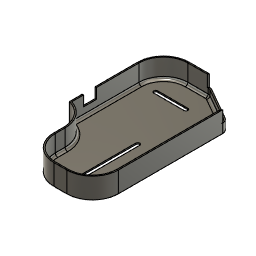
case (Autodesk Fusion 360 design; units mm, degrees)
Autodesk Fusion 360 part; units mm, degrees
note: some values were not read from the file. Chosen so that the rebuilt part matches the saved one: a direction.
sketch "Sketch1" plane through (0, 0, 0) normal (0, 1, 0) x (1, 0, 0)
  line L0 (-0.1777, 0.064) -> (49.8223, 0.064)
  line L1 (49.8223, 0.064) -> (49.8223, -119.936)
  line L2 (49.8223, -119.936) -> (-0.1777, -119.936)
  line L3 (-0.1777, -119.936) -> (-0.1777, 0.064)
  line L4 (-0.1777, 0.064) -> (-15.1777, 0.064)
  line L5 (-15.1777, 0.064) -> (-15.1777, -72.936)
  line L6 (-15.1777, -72.936) -> (-0.1777, -72.936)
  line L7 (-0.1777, -72.936) -> (-0.1777, 0.064)
  dimension "d1" = 50
  dimension "d2" = 120
  dimension "d3" = 15
  dimension "d4" = 73
  constraint horizontal L0
  constraint vertical L1
  constraint horizontal L2
  constraint vertical L3
  constraint horizontal L4
  constraint vertical L5
  constraint horizontal L6
  constraint vertical L7
  measures "d1" distance of L0.start L0.end
  measures "d2" distance of L0.start L2.end
  measures "d3" distance of L0.start L4.end
  measures "d4" distance of L0.start L6.end
extrude "Extrude1" add sketch "Sketch1" along normal blind 2
fillet "Fillet1" radius 20 4 edges at (-0.1777, 1, 72.936) (-0.1777, 1, 119.936) (49.8223, 1, 119.936) (-15.1777, 1, -0.064)
sketch "Sketch2" plane through (0, 2, 0) normal (0, 1, 0) x (-1, 0, 0)
  arc A0 (-4.8223, -0.064) -> (15.1777, 19.936) centre (-4.8223, 19.936) ccw
  line L0 (15.1777, 19.936) -> (15.1777, 72.936)
  arc A1 (0.1777, 92.3009) -> (15.1777, 72.936) centre (20.1777, 92.3009) ccw
  line L1 (0.1777, 92.3009) -> (0.1777, 99.936)
  arc A2 (0.1777, 99.936) -> (-19.8223, 119.936) centre (-19.8223, 99.936) ccw
  line L2 (-19.8223, 119.936) -> (-29.8223, 119.936)
  arc A3 (-29.8223, 119.936) -> (-49.8223, 99.936) centre (-29.8223, 99.936) ccw
  line L3 (-49.8223, 99.936) -> (-49.8223, -0.064)
  line L4 (-49.8223, -0.064) -> (-4.8223, -0.064)
  line L5 (-21.8223, -0.064) -> (-49.8223, 15.936)
  dimension "d9" = 28
  dimension "d10" = 16
  constraint coincident L4 L5.start
  constraint coincident L3 L5.end
  measures "d9" distance of L3.end L5.start
  measures "d10" distance of L3.end L5.end
extrude "Extrude2" cut sketch "Sketch2" against normal blind 2 contours L3 L4 L5
fillet "Fillet2" radius 5 2 edges at (49.8223, 1, 15.936) (21.8223, 1, -0.064)
extrude "Extrude3" add 1 faces at (32.044, 2, 66.6722) along direction (0, 1, 0) blind 14
shell "Shell1" thickness 1 removed faces 1 at (32.044, 16, 66.6722)
sketch "Sketch3" plane through (5.3992, 0, -9.4486) normal (0.496139, 0, -0.868243) x (-0.868243, 0, -0.496139)
  line L0 (-20.2431, 0) -> (-20.2431, 16)
  line L1 (-20.2431, 16) -> (-48.2627, 16)
  line L2 (-48.2627, 16) -> (-48.2627, 0)
  line L3 (-48.2627, 0) -> (-20.2431, 0)
  line L4 (-52.6039, 16) -> (-17.7624, 16)
  line L5 (-17.7624, 16) -> (-17.7624, 7)
  line L6 (-17.7624, 7) -> (-52.6039, 7)
  line L7 (-52.6039, 7) -> (-52.6039, 16)
  line L8 (-52.6039, 16) -> (-52.6039, 0)
  line L9 (-17.7624, 0) -> (-17.7624, 16)
  dimension "d18" = 9
  constraint horizontal L4
  constraint vertical L5
  constraint horizontal L6
  constraint vertical L7
  constraint collinear L1 L4
  constraint collinear L7 L8
  constraint collinear L5 L9
  measures "d18" distance of L4 L6
extrude "Extrude4" cut sketch "Sketch3" against normal blind 5 contours L0 L1 L2 L4 L6 | L0 L4 L5 L6 L9 | L2 L4 L6 L7 L8
sketch "Sketch4" plane through (-15.1777, 0, 0) normal (-1, 0, 0) x (0, 0, 1)
  line L0 (19.936, 16) -> (19.936, 0)
  line L1 (19.936, 0) -> (72.936, 0)
  line L2 (72.936, 0) -> (72.936, 16)
  line L3 (72.936, 16) -> (19.936, 16)
  line L4 (52.936, 16) -> (62.936, 16)
  line L5 (62.936, 16) -> (62.936, 8)
  line L6 (62.936, 8) -> (52.936, 8)
  line L7 (52.936, 8) -> (52.936, 16)
  line L8 (-0.064, 7) -> (-0.064, 16)
  dimension "d21" = 8
  dimension "d22" = 10
  dimension "d23" = 53
  constraint horizontal L4
  constraint vertical L5
  constraint horizontal L6
  constraint vertical L7
  constraint collinear L3 L4
  measures "d21" distance of L4.end L5.end
  measures "d22" distance of L5.end L6.end
  measures "d23" distance of L4.start L8.end
extrude "Extrude5" cut sketch "Sketch4" against normal blind 1 contours L3 L4 L5 L6 L7
fillet "Fillet3" radius 2 12 edges at (-14.1777, 1, 46.0562) (-8.6127, 1, 6.501) (12.6584, 1, 0.936) (21.5211, 1, 1.07) (34.6429, 1, 8.4138) (48.2819, 1, 16.8299) (48.8223, 1, 59.3868) (43.2573, 1, 113.371) (24.8223, 1, 118.936) (6.3873, 1, 113.371) (0.8223, 1, 96.1185) (-3.3403, 1, 79.751)
sketch "Sketch5" plane through (0, 1, 0) normal (0, 1, 0) x (-1, 0, 0)
  arc A0 (-2.8223, 92.3009) -> (12.1777, 70.7371) centre (20.1777, 92.3009) ccw
  line L0 (-2.8223, 92.3009) -> (-2.8223, 99.936)
  arc A1 (-2.8223, 99.936) -> (-19.8223, 116.936) centre (-19.8223, 99.936) ccw
  line L1 (-19.8223, 116.936) -> (-29.8223, 116.936)
  arc A2 (-29.8223, 116.936) -> (-46.8223, 99.936) centre (-29.8223, 99.936) ccw
  line L2 (-46.8223, 99.936) -> (-46.8223, 18.8376)
  arc A3 (-46.8223, 18.8376) -> (-45.8146, 17.1011) centre (-44.8223, 18.8376) ccw
  line L3 (-45.8146, 17.1011) -> (-21.4867, 3.1995)
  arc A4 (-21.4867, 3.1995) -> (-20.4945, 2.936) centre (-20.4945, 4.936) ccw
  line L4 (-20.4945, 2.936) -> (-4.8223, 2.936)
  arc A5 (-4.8223, 2.936) -> (12.1777, 19.936) centre (-4.8223, 19.936) ccw
  line L5 (12.1777, 19.936) -> (12.1777, 70.7371)
  line L6 (3.1494, 19.436) -> (-20.2783, 19.436)
  arc A6 (-20.2783, 19.436) -> (-20.2783, 16.436) centre (-20.2783, 17.936) ccw
  line L7 (-20.2783, 16.436) -> (3.1494, 16.436)
  arc A7 (3.1494, 16.436) -> (3.1494, 19.436) centre (3.1494, 17.936) ccw
  line L8 (3.1494, 17.936) -> (-20.2783, 17.936) construction
  line L9 (-20.4945, -0.064) -> (-4.8223, -0.064)
  line L10 (-23.5, 60) -> (-23.5, 110)
  arc A8 (-23.5, 110) -> (-26.5, 110) centre (-25, 110) ccw
  line L11 (-26.5, 110) -> (-26.5, 60)
  arc A9 (-26.5, 60) -> (-23.5, 60) centre (-25, 60) ccw
  line L12 (-25, 60) -> (-25, 110) construction
  dimension "d28" = 3
  dimension "d29" = 16.5
  dimension "d30" = 3
  constraint tangent L6 A6
  constraint tangent A6 L7
  constraint parallel L6 L7
  constraint tangent L7 A7
  constraint tangent L6 A7
  constraint horizontal L8
  constraint tangent L10 A8
  constraint tangent A8 L11
  constraint parallel L10 L11
  constraint tangent L11 A9
  constraint tangent L10 A9
  constraint parallel L5 L12
  measures "d28" diameter of A6
  measures "d29" distance of L7 L9
  measures "d30" diameter of A8
extrude "Extrude6" cut sketch "Sketch5" against normal blind 2 contours L6 A6 L7 A7 | L10 A8 L11 A9
